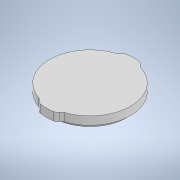
# Autodesk Inventor part: HSI cap
Saved by Autodesk Inventor 2022 (Build 260153000, 153)
## iProperties
Created: 2022-03-31
Part Number: HSI cap
Material: Generic
Document SubType Name: Modeling
Designer: RNG3nius
Density: 1 g/cm^3
Appearance: Default
Author: RNG3nius
Autodesk Inventor part; units mm, degrees
ref_plane "YZ Plane" through (0, 0, 0) normal (1, 0, 0) x (0, 1, 0)
ref_plane "XZ Plane" through (0, 0, 0) normal (0, 1, 0) x (-1, 0, 0)
ref_plane "XY Plane" through (0, 0, 0) normal (0, 0, 1) x (1, 0, 0)
sketch "Sketch1" plane through (0, 0, 0) normal (0, 1, 0) x (-1, 0, 0)
  circle A0 centre (0, 0) radius 25.725
  dimension "d0" = 51.45
  constraints: 1 centre point, 1 coincident
  measures "d0" diameter of A0
extrude "Extrusion1" add sketch "Sketch1" along normal blind 3
sketch "Sketch2" plane through (0, 3, 0) normal (0, 1, 0) x (1, 0, 0)
  circle A0 centre (0, 0) radius 28.8
  dimension "d3" = 57.6
  constraints: 1 centre point, 1 coincident
  measures "d3" diameter of A0
extrude "Extrusion2" add sketch "Sketch2" along normal blind 5.8
sketch "Sketch5" plane through (0, 3, 0) normal (0, -1, 0) x (1, 0, 0)
  circle A0 centre (0, 0) radius 28.8 projected
  line L0 (8, -27.6666) -> (6.5, -30.2647)
  line L1 (8, -27.6666) -> (11, -27.6666) construction
  line L2 (-8, -27.6666) -> (-6.5, -30.2647)
  line L3 (-8, -27.6666) -> (-5, -27.6666) construction
  arc A1 (-6.5, -30.2647) -> (6.5, -30.2647) centre (0, -2.2078) ccw
  dimension "d33" = 16
  dimension "d34" = 27.6666
  dimension "d35" = 27.6666
  dimension "d36" = 3
  dimension "d37" = 120
  dimension "d38" = 3
  dimension "d39" = 60
  dimension "d40" = 28.8
  constraints: 8 end point, 2 equal length, 2 horizontal, 2 point on circle, 1 centre point, 2 other
  measures "d33" distance of L2.start L0.start
  measures "d34" vertical distance of point (0, 0) L2.start
  measures "d35" vertical distance of point (0, 0) L0.start
  measures "d36" distance of L0.start L0.end
  measures "d37" angle of L0 L1
  measures "d38" distance of L2.start L2.end
  measures "d39" angle of L2 L3
  measures "d40" radius of A1
extrude "Extrusion4" add sketch "Sketch5" against normal up to surface (5.8 mm away) contours A0 L0 A1 L2
fillet "Fillet2" radius 4 4 edges at (8, 5.9, -27.6666) (6.5, 5.9, -30.2647) (-6.5, 5.9, -30.2647) (-8, 5.9, -27.6666)
pattern_circular "Circular Pattern1" count 2 over 360 about axis through (0, 3, 0) along (0, 1, 0) of "Extrusion4", "Fillet2"
sketch "Sketch6" plane through (0, 0, 0) normal (0, 0, 1) x (1, 0, 0)
  line L0 (-25.725, 0) -> (-25.725, 3) projected
  line L1 (-25.725, 3) -> (-28.8, 3)
  line L2 (-28.8, 3) -> (-28.8, 1)
  line L3 (-28.8, 1) -> (-25.725, 1)
  line L4 (-25.725, 1) -> (-25.725, 3)
  line L5 (25.725, 0) -> (-25.725, 0) projected
  line L6 (0, -0.6) -> (0, 3.6) projected
  point P0 (0, 0)
  dimension "d44" = 3.075
  dimension "d45" = 2
  dimension "d46" = 1
  constraints: 8 end point, 2 parallel, 1 horizontal, 1 perpendicular, 1 point on line
  measures "d44" distance of L3.end L2.end
  measures "d45" distance of L2.end L1.end
  measures "d46" distance between parallel lines of L5 L3
revolve "Revolution1" add sketch "Sketch6" angle 12.51 about axis through (0, -10, 0) along (0, 1, 0) and the other way 12.51
fillet "Fillet3" radius 0.5 2 edges at (-26.6152, 1, 5.9053) (-26.6152, 1, -5.9053)
body "Solid1"
